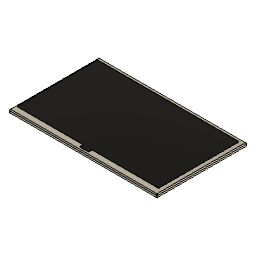
Omni-Cube (Autodesk Fusion 360 archive; units mm, degrees)
design "7  Displat PID 2353"
Autodesk Fusion 360 part; units mm, degrees
sketch "Sketch1" plane through (0, 0, 0) normal (0, 0, 1) x (1, 0, 0) in component "Display"
  line L0 (0, 0) -> (164, 0)
  line L1 (164, 0) -> (164, 100)
  line L2 (164, 100) -> (0, 100)
  line L3 (0, 100) -> (0, 0)
  dimension "d1" = 164
  dimension "d2" = 100
  constraint horizontal L0
  constraint vertical L1
  constraint horizontal L2
  constraint vertical L3
  constraint coincident L0.start L3.end
  measures "d1" distance of L0.start L0.end
  measures "d2" distance of L0.start L2.end
extrude "Extrude1" add sketch "Sketch1" along normal blind 4 in component "Display"
fillet "Fillet1" radius 1 12 edges at (164, 100, 2) (164, 50, 0) (82, 100, 4) (0, 0, 2) (164, 50, 4) (0, 50, 4) (82, 0, 4) (82, 0, 0) (0, 50, 0) (164, 0, 2) (82, 100, 0) (0, 100, 2) in component "Display"
sketch "Sketch2" plane through (0, 0, 4) normal (0, 0, 1) x (-1, 0, 0) in component "Display"
  line L0 (-163, -99) -> (-1, -99)
  line L1 (-1, -99) -> (-1, -1)
  line L2 (-1, -1) -> (-163, -1)
  line L3 (-163, -1) -> (-163, -99)
  line L4 (-1.81, -96.43) -> (-158.51, -96.43)
  line L5 (-158.51, -96.43) -> (-158.51, -7.33)
  line L6 (-158.51, -7.33) -> (-1.81, -7.33)
  line L7 (-1.81, -7.33) -> (-1.81, -96.43)
  line L8 (-164, -100) -> (0, -100)
  line L9 (-164, 0) -> (-164, -100)
  line L10 (-75.16, -7.33) -> (-85.16, -7.33)
  line L11 (-85.16, -7.33) -> (-85.16, -3.33)
  line L12 (-85.16, -3.33) -> (-75.16, -3.33)
  line L13 (-75.16, -3.33) -> (-75.16, -7.33)
  line L14 (-80.16, -3.33) -> (-80.16, -7.33) construction
  dimension "d7" = 3.57
  dimension "d8" = 5.49
  dimension "d9" = 156.7
  dimension "d10" = 89.1
  dimension "d13" = 10
  dimension "d14" = 4
  constraint horizontal L4
  constraint vertical L5
  constraint horizontal L6
  constraint vertical L7
  constraint horizontal L10
  constraint vertical L11
  constraint horizontal L12
  constraint vertical L13
  constraint coincident L6 L10.start
  constraint midpoint L12 L14.start
  constraint midpoint L10 L14.end
  constraint midpoint L6 L14.end
  measures "d7" distance of L4 L8
  measures "d8" distance of L5 L9
  measures "d9" distance of L4.start L4.end
  measures "d10" distance of L4.start L6.end
  measures "d13" distance of L11.end L12.end
  measures "d14" distance of L10.end L11.end
extrude "Extrude2" cut sketch "Sketch2" against normal blind 0.2 contours L4 L5 L6 L7 L10 | L6 L10 L11 L12 L13 in component "Display"
component "Display" placed x (1, 0, 0) y (0, 1, 0) z (0, 0, 1) at (0, 0, 0)
